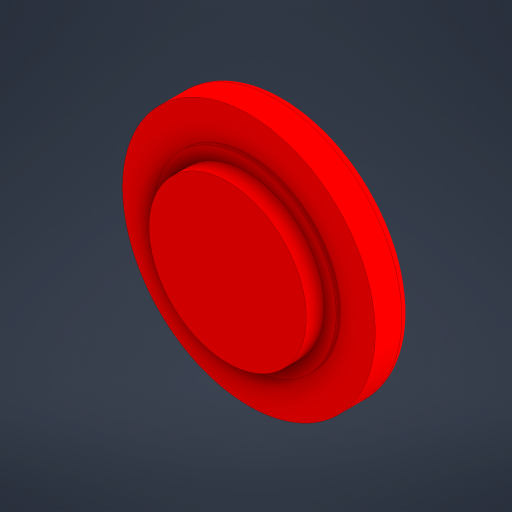
# Autodesk Inventor part: Outer Ring Press
Saved by Autodesk Inventor 2023.4 (Build 274418000, 418)
## iProperties
Created: 2024-07-23
Part Number: Outer Ring Press
Material: Generic
Document SubType Name: Modeling
Designer: xSibe
Density: 1 g/cm^3
Appearance: Plastic Red
Author: xSibe
Autodesk Inventor part; units mm, degrees
ref_plane "YZ Plane" through (0, 0, 0) normal (1, 0, 0) x (0, 1, 0)
ref_plane "XZ Plane" through (0, 0, 0) normal (0, 1, 0) x (-1, 0, 0)
ref_plane "XY Plane" through (0, 0, 0) normal (0, 0, 1) x (1, 0, 0)
sketch "Sketch1" plane through (0, 0, 0) normal (0, 0, 1) x (1, 0, 0)
  circle A0 centre (0, 0) radius 11.125
  circle A1 centre (0, 0) radius 12.875
  circle A2 centre (0, 0) radius 17.875
  dimension "d0" = 22.25
  dimension "d1" = 25.75
  dimension "d2" = 5
  constraints: 3 centre point, 2 coincident
  measures "d0" diameter of A0
  measures "d1" diameter of A1
  measures "d2" radial gap between concentric circles of A1 A2
extrude "Extrusion1" add sketch "Sketch1" along normal blind 5 contours A0 | A1 | A2
extrude "Extrusion2" add sketch "Sketch1" along normal blind 0.5 from surface at 5 contours A0 | A1
extrude "Extrusion3" add sketch "Sketch1" along normal blind 2.5 from surface at 5.5 contours A0
fillet "Fillet1" radius 1.25 1 edges at (-17.875, 0, 0)
sketch "Sketch2" plane through (0, 0, 0) normal (0, 0, -1) x (-1, 0, 0)
  line L0 (-12.5, -12.5) -> (12.5, -12.5)
  line L1 (12.5, -12.5) -> (12.5, 12.5)
  line L2 (12.5, 12.5) -> (-12.5, 12.5)
  line L3 (-12.5, 12.5) -> (-12.5, -12.5)
  line L4 (-12.5, -12.5) -> (12.5, 12.5) construction
  line L5 (12.5, -12.5) -> (-12.5, 12.5) construction
  line L6 (-12.5, 12.5) -> (12.5, 12.5) construction
  line L7 (12.5, 12.5) -> (12.5, -12.5) construction
  line L8 (12.5, -12.5) -> (-12.5, -12.5) construction
  line L9 (-12.5, -12.5) -> (-12.5, 12.5) construction
  spline S0 degree 2 poles (6.4425, 7.7147) (7.577, 6.3857) (8.8412, 2.4959) (8.8412, 0) knots 0 0 0 1 2 2 2
  spline S1 degree 2 poles (8.8412, 0) (8.8412, -2.4311) (7.6094, -6.3695) (6.4425, -7.6985) knots 0 0 0 1 2 2 2
  spline S2 degree 2 poles (6.4425, -7.6985) (5.2107, -9.0924) (1.953, -10.4214) (-0.0081, -10.4214) knots 0 0 0 1 2 2 2
  spline S3 degree 2 poles (-0.0081, -10.4214) (-2.034, -10.4214) (-5.2755, -9.0438) (-6.4587, -7.6985) knots 0 0 0 1 2 2 2
  spline S4 degree 2 poles (-6.4587, -7.6985) (-7.6094, -6.3695) (-8.8412, -2.4635) (-8.8412, 0) knots 0 0 0 1 2 2 2
  spline S5 degree 2 poles (-8.8412, 0) (-8.8412, 2.5122) (-7.5932, 6.3371) (-6.4425, 7.7147) knots 0 0 0 1 2 2 2
  spline S6 degree 2 poles (-6.4425, 7.7147) (-5.2755, 9.0438) (-2.0178, 10.4214) (-0.0081, 10.4214) knots 0 0 0 1 2 2 2
  spline S7 degree 2 poles (-0.0081, 10.4214) (2.034, 10.4214) (5.3079, 8.9951) (6.4425, 7.7147) knots 0 0 0 1 2 2 2
  spline S8 degree 2 poles (6.0697, 0) (6.0697, 1.9773) (5.2107, 5.0405) (4.4327, 6.0454) knots 0 0 0 1 2 2 2
  spline S9 degree 2 poles (4.4327, 6.0454) (3.6386, 7.0827) (1.4019, 8.1199) (0.0081, 8.1199) knots 0 0 0 1 2 2 2
  spline S10 degree 2 poles (0.0081, 8.1199) (-1.4344, 8.1199) (-3.6062, 7.1151) (-4.4327, 6.0454) knots 0 0 0 1 2 2 2
  spline S11 degree 2 poles (-4.4327, 6.0454) (-5.2269, 5.0243) (-6.0697, 1.9449) (-6.0697, 0) knots 0 0 0 1 2 2 2
  spline S12 degree 2 poles (-6.0697, 0) (-6.0697, -3.9384) (-2.7634, -8.1199) (0.0081, -8.1199) knots 0 0 0 1 2 2 2
  spline S13 degree 2 poles (0.0081, -8.1199) (2.7796, -8.1199) (6.0697, -3.9384) (6.0697, 0) knots 0 0 0 1 2 2 2
  point P0 (0, 0)
  dimension "d10" = 25
  dimension "d11" = 25
  constraints: 12 end point, 2 coincident, 2 midpoint, 2 parallel, 1 horizontal, 1 perpendicular, 2 other
  measures "d10" distance of L2.end L1.end
  measures "d11" distance of L1.end L0.end
extrude "Extrusion4" cut sketch "Sketch2" against normal blind 0.25 contours S0 S1 S2 S3 S4 S5 S6 S7
chamfer "Chamfer1" distance 0.25 angle 45 14 edges at (-8.2091, 4.4408, 0.25) (-8.2253, -4.4003, 0.25) (-3.5818, -9.7569, 0.25) (3.6548, -9.7326, 0.25) (8.2253, -4.4165, 0.25) (8.2172, 4.4246, 0.25) (3.6467, 9.7326, 0.25) (-3.671, 9.7083, 0.25) (-4.4246, -6.0292, 0.25) (-5.6402, 3.5089, 0.25) (-2.5203, 7.6013, 0.25) (2.5203, 7.6175, 0.25) (5.6483, 3.4846, 0.25) (4.4165, -6.0292, 0.25)
body "Solid1"
